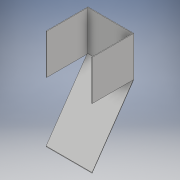
# Autodesk Inventor part: Ramp
Saved by Autodesk Inventor 2018 (Build 220112000, 112)
## iProperties
Created: 2017-04-15
Part Number: Ramp
Material: Generic
Document SubType Name: Modeling
Designer: Administrator
Density: 1 g/cm^3
Appearance: Default
Author: Administrator
Autodesk Inventor part; units mm, degrees
ref_plane "YZ Plane" through (0, 0, 0) normal (1, 0, 0) x (0, 1, 0)
ref_plane "XZ Plane" through (0, 0, 0) normal (0, 1, 0) x (-1, 0, 0)
ref_plane "XY Plane" through (0, 0, 0) normal (0, 0, 1) x (1, 0, 0)
sketch "Sketch1" plane through (0, 0, 0) normal (0, 0, 1) x (1, 0, 0)
  line L0 (0, 0) -> (0, 70)
  line L1 (0, 70) -> (77, 70)
  line L2 (77, 70) -> (77, 0)
  line L3 (0, 0) -> (1, 0)
  line L4 (1, 0) -> (1, 69)
  line L5 (1, 69) -> (76, 69)
  line L6 (76, 69) -> (76, 0)
  line L7 (76, 69) -> (145, 69) construction
  line L8 (76, 0) -> (76, 1)
  line L9 (76, 0) -> (77, 0)
  dimension "d0" = 70
  dimension "d1" = 77
  dimension "d3" = 70
  dimension "d5" = 1
  dimension "d6" = 69
  dimension "d7" = 90
  dimension "d8" = 75
  dimension "d9" = 90
  dimension "d10" = 69
  dimension "d11" = 90
  dimension "d12" = 1
  constraints: 20 end point, 6 perpendicular, 1 horizontal, 1 parallel, 1 point on line, 1 vertical
  measures "d0" distance of L0.start L0.end
  measures "d1" distance of L0.end L1.end
  measures "d3" distance of L1.end L2.end
  measures "d5" distance of L0.start L3.end
  measures "d6" distance of L3.end L4.end
  measures "d7" angle of L4 L3
  measures "d8" distance of L4.end L5.end
  measures "d9" angle of L4 L5
  measures "d10" distance of L5.end L6.end
  measures "d11" angle of L6 L7
  measures "d12" distance of L6.end L8.end
extrude "Extrusion1" add sketch "Sketch1" along normal blind 67
sketch "Sketch2" plane through (77, 0, 0) normal (1, 0, 0) x (0, 0, -1)
  line L0 (0, 70) -> (-67, 70) projected
  line L1 (0, 70) -> (0, 69)
  line L2 (0, 70) -> (1, 70) construction
  line L3 (100, 0) -> (101, 0)
  line L4 (100, 0) -> (101, 0) construction
  line L5 (101, 0) -> (0, 70)
  line L6 (100, 0) -> (0, 69)
  point P0 (0, 0)
  dimension "d15" = 1
  dimension "d16" = 90
  dimension "d17" = 1
  dimension "d18" = 0
  constraints: 12 end point, 3 horizontal, 2 equal length, 1 vertical
  measures "d15" distance of L0.start L1.end
  measures "d16" angle of L1 L2
  measures "d17" distance of L3.start L3.end
  measures "d18" distance between parallel lines of L3 L4
extrude "Extrusion2" add sketch "Sketch2" against normal blind 77
body "Solid1"
